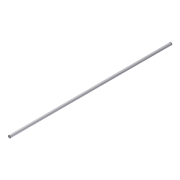
# Autodesk Inventor part: FE-00004-02C
Saved by Autodesk Inventor 2012 (Build 160160000, 160)
## iProperties
Created: 2008-05-29
Part Number: FE-00004-02C
Document SubType Name: Modeling
Designer: narosenberg
Density: 1 g/cm^3
Mass: 12.8704 g
Surface Area: 81.7066 cm^2
Volume: 12.8704 cm^3
Material: Default
Author: narosenberg
Autodesk Inventor part; units mm, degrees
ref_plane "XZ Plane" through (0, 0, 0) normal (0, 1, 0) x (-1, 0, 0)
ref_plane "XY Plane" through (0, 0, 0) normal (0, 0, 1) x (1, 0, 0)
sketch "Sketch1" plane through (0, 0, 0) normal (0, 0, 1) x (1, 0, 0)
  circle A0 centre (-18.0818, 12.1069) radius 3.175
  dimension "d0" = 6.35
  constraints: 1 centre point
  measures "d0" diameter of A0
extrude "Extrusion1" add sketch "Sketch1" along normal blind 406.4
ref_plane "Work Plane1" through (-18.0818, 12.1069, 0) normal (0, 1, 0) x (0, 0, 1)
body "Solid1"
